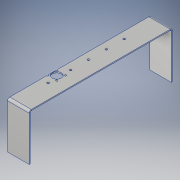
# Autodesk Inventor part: Turret Support Brace
Saved by Autodesk Inventor 2019.4 (Build 234330000, 330)
## iProperties
Created: 2020-01-12
Part Number: Turret Support Brace
Material: Aluminum 6061
Document SubType Name: Sheet Metal
Designer: admin
Density: 2.7 g/cm^3
Sheet Metal Rule: Default_mm
Appearance: Aluminum - Flat
Author: admin
Autodesk Inventor part; units mm, degrees
ref_plane "YZ Plane" through (0, 0, 0) normal (1, 0, 0) x (0, 1, 0)
ref_plane "XZ Plane" through (0, 0, 0) normal (0, 1, 0) x (-1, 0, 0)
ref_plane "XY Plane" through (0, 0, 0) normal (0, 0, 1) x (1, 0, 0)
sketch "Sketch1" plane through (0, 0, 0) normal (0, 1, 0) x (-1, 0, 0)
  line L0 (-30, 200) -> (30, 200)
  line L1 (30, 200) -> (30, -200)
  line L2 (30, -200) -> (-30, -200)
  line L3 (-30, -200) -> (-30, 200)
  line L4 (-30, 200) -> (30, -200) construction
  line L5 (30, 200) -> (-30, -200) construction
  point P0 (0, 0)
  dimension "d0" = 60
  dimension "d1" = 400
  measures "d0" distance of L1.end L2.end
  measures "d1" distance of L0.end L1.end
extrude "Plate1" add sketch "Sketch1" along normal blind 3
sketch "Sketch2" plane through (-30, 3, 197) normal (0, 0, 1) x (1, 0, 0)
  line L0 (60, 0) -> (0, 0)
  line L1 (0, 0) -> (0, -130)
  line L2 (0, -130) -> (60, -130)
  line L3 (60, -130) -> (60, 0)
  constraints: 6 end point, 1 horizontal, 1 perpendicular, 1 vertical
edge flange "Flange1" height 130 angle 90 thickness 3 bend radius 3 thickness toward (0, 0, 1) relief straight relief width 3 relief depth 1.5 corner gap 3 corner form 0 edges at (0, 0, 200) (0, 0, -200) wall of the first edge with corners at (30, 3, 197) (-30, 3, 197) (-30, -127, 197) (30, -127, 197)
bend "Bend1"
corner "Corner1"
sketch "Sketch3" plane through (0, 3, 0) normal (0, 1, 0) x (1, 0, 0)
  circle A0 centre (-10.5, -106.3097) radius 2.75 projected
  circle A1 centre (-10.5, -43.6903) radius 2.75 projected
  circle A2 centre (-4.3429, -88.5614) radius 2.25 projected
  circle A3 centre (-4.3429, -63.8126) radius 2.25 projected
  circle A4 centre (-29.0916, -88.5614) radius 2.25 projected
  circle A5 centre (-29.0916, -63.8126) radius 2.25 projected
  circle A6 centre (-10.5, 6.3097) radius 2.75 projected
  circle A7 centre (-10.5, 56.3097) radius 2.75 projected
  circle A8 centre (-10.5, 106.3097) radius 2.75 projected
  circle A9 centre (-16.7173, -76.187) radius 12.75 projected
  point P0 (0, 0)
extrude "Extrusion1" cut sketch "Sketch3" against normal through all
fillet "Fillet1" radius 3 4 edges at (-30, 1.5, 90.6199) (-30, 1.5, 86.5029) (-30, 1.5, 65.8711) (-30, 1.5, 61.7541)
equation "\"d2\" = Thickness"
equation "\"d3\" = BendReliefWidth"
equation "\"d4\" = BendReliefDepth"
equation "\"d5\" = MinimumRemnant"
equation "\"d6\" = TransitionRadius"
equation "\"d9\" = BendRadius"
equation "\"d10\" = CornerReliefSize"
equation "\"d11\" = GapSize"
equation "\"d12\" = JacobiRadiusSize"
equation "\"BendRadius\" = Thickness"
equation "\"BendReliefWidth\" = Thickness"
equation "\"BendReliefDepth\" = 0.5 * Thickness"
equation "\"CornerReliefSize\" = 4 * Thickness"
equation "\"MinimumRemnant\" = 2 * Thickness"
equation "\"TransitionRadius\" = BendRadius"
equation "\"JacobiRadiusSize\" = BendRadius"
equation "\"GapSize\" = Thickness"
equation "\"Thickness\" = 3"
body "Solid1"
